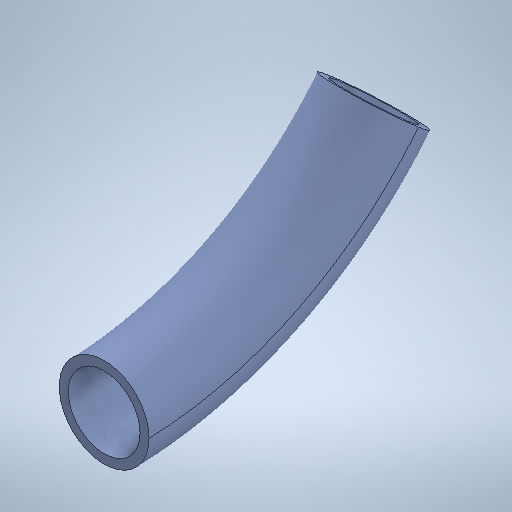
# Autodesk Inventor part: peca_004_001
Saved by Autodesk Inventor 2025.2 (Build 292293000, 293)
## iProperties
Created: 2025-03-25
Part Number: peca_004_001
Material: Borracha
Document SubType Name: Modeling
Designer: Carlos Dias
Density: 0.93 g/cm^3
Appearance: Borracha - Azul
Author: Carlos Dias
Autodesk Inventor part; units mm, degrees
ref_plane "YZ Plane" through (0, 0, 0) normal (1, 0, 0) x (0, 1, 0)
ref_plane "XZ Plane" through (0, 0, 0) normal (0, 1, 0) x (-1, 0, 0)
ref_plane "XY Plane" through (0, 0, 0) normal (0, 0, 1) x (1, 0, 0)
sketch "Esboço1" plane through (0, 0, 0) normal (0, 0, 1) x (1, 0, 0)
  circle A0 centre (0, 0) radius 5
  circle A1 centre (0, 0) radius 4
  dimension "d0" = 10
  dimension "d1" = 1
  constraints: 2 centre point, 2 coincident
  measures "d0" diameter of A0
  measures "d1" radial gap between concentric circles of A0 A1
sketch "Esboço2" plane through (0, 0, 0) normal (1, 0, 0) x (0, 1, 0)
  arc A0 (0, 0) -> (15, -30) centre (39.9808, 1.2404) ccw
  dimension "d2" = 40
  dimension "d6" = 30
  dimension "d7" = 15
  constraints: 2 point on circle, 1 centre point, 1 coincident
  measures "d2" radius of A0
  measures "d6" vertical distance of A0.end point (0, 0)
  measures "d7" horizontal distance of A0.end point (0, 0)
sweep "Varredura1" add profiles "Esboço1" path "Esboço2"
